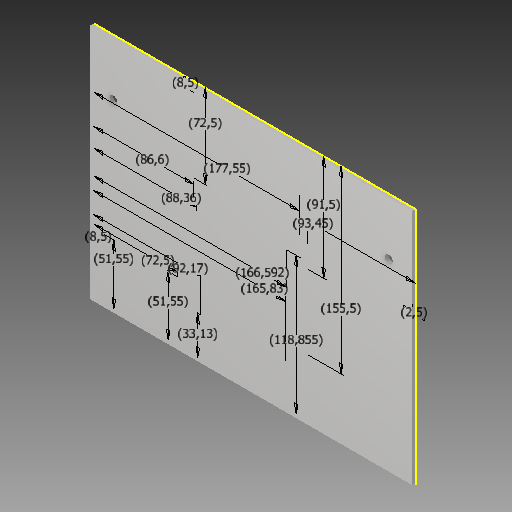
# Autodesk Inventor part: SupportsheetADCS2
Saved by Autodesk Inventor 2017 (Build 210142000, 142)
## iProperties
Created: 2016-11-08
Part Number: SupportsheetADCS2
Material: Aluminum 6061
Document SubType Name: Modeling
Designer: Jonis
Density: 2.7 g/cm^3
Appearance: Aluminum - Flat
Author: Jonis
Autodesk Inventor part; units mm, degrees
ref_plane "YZ Plane" through (0, 0, 0) normal (1, 0, 0) x (0, 1, 0)
ref_plane "XZ Plane" through (0, 0, 0) normal (0, 1, 0) x (-1, 0, 0)
ref_plane "XY Plane" through (0, 0, 0) normal (0, 0, 1) x (1, 0, 0)
sketch "Sketch1" plane through (0, 0, 0) normal (0, 0, 1) x (1, 0, 0)
  line L0 (0, 0) -> (278, 0)
  line L1 (278, 0) -> (278, 179)
  line L2 (278, 179) -> (0, 179)
  line L3 (0, 179) -> (0, 0)
  dimension "d0" = 278
  dimension "d1" = 179
  constraints: 8 end point, 2 parallel, 1 horizontal, 1 perpendicular
  measures "d0" distance of L2.end L1.end
  measures "d1" distance of L1.end L0.end
extrude "Extrusion1" add sketch "Sketch1" along normal blind 3
sketch "Sketch2" plane through (0, 0, 3) normal (0, 0, 1) x (1, 0, 0)
  line L0 (0, 179) -> (0, 0) projected
  line L1 (278, 179) -> (0, 179) projected
  line L2 (278, 0) -> (278, 179) projected
  point P0 (20, 159)
  point P1 (258, 159)
  dimension "d4" = 20
  dimension "d5" = 20
  dimension "d6" = 20
  dimension "d7" = 20
  measures "d4" distance from line of L0 point (20, 159)
  measures "d5" distance from line of L1 point (20, 159)
  measures "d6" distance from line of L1 point (258, 159)
  measures "d7" distance from line of L2 point (258, 159)
hole "Hole1" at (20, 159, 3) at (258, 159, 3) direction (0, 0, -1) diameter 7 end through all
sketch "Sketch6" plane through (0, 179, 0) normal (0, 1, 0) x (1, 0, 0)
  line L0 (0, 0) -> (278, 0) projected
  line L1 (0, -3) -> (278, -3) projected
  line L2 (0, 0) -> (278, 0)
  line L3 (278, 0) -> (278, -3)
  line L4 (278, -3) -> (0, -3)
  line L5 (0, -3) -> (0, 0)
  constraints: 8 end point, 2 parallel, 1 horizontal, 1 perpendicular
extrude "Extrusion2" add sketch "Sketch6" along normal blind 26
sketch "Sketch7" plane through (0, 0, 0) normal (0, 0, -1) x (-1, 0, 0)
  circle A0 centre (-92.17, 33.13) radius 1.5875 projected
  circle A1 centre (-165.83, 33.13) radius 1.5875 projected
  circle A2 centre (-166.592, 118.855) radius 1.5875 projected
  circle A3 centre (-88.36, 118.855) radius 1.5875 projected
  circle A4 centre (-8.5, 51.55) radius 1.6 projected
  circle A5 centre (-72.5, 51.55) radius 1.6 projected
  circle A6 centre (-72.5, 142.5) radius 1.6 projected
  circle A7 centre (-8.5, 142.5) radius 1.6 projected
  circle A8 centre (-86.6, 132.5) radius 1.6 projected
  circle A9 centre (-86.6, 196.5) radius 1.6 projected
  circle A10 centre (-177.55, 196.5) radius 1.6 projected
  circle A11 centre (-177.55, 132.5) radius 1.6 projected
  circle A12 centre (-184.55, 132.5) radius 1.6 projected
  circle A13 centre (-184.55, 196.5) radius 1.6 projected
  circle A14 centre (-275.5, 196.5) radius 1.6 projected
  circle A15 centre (-275.5, 132.5) radius 1.6 projected
  circle A16 centre (-275.5, 113.5) radius 1.6 projected
  circle A17 centre (-275.5, 49.5) radius 1.6 projected
  circle A18 centre (-184.55, 49.5) radius 1.6 projected
  circle A19 centre (-184.55, 113.5) radius 1.6 projected
  line L0 (0, 0) -> (-278, 0) projected
  line L1 (0, 0) -> (0, 205) projected
  line L2 (-278, 205) -> (0, 205) projected
  line L3 (-278, 0) -> (-278, 205) projected
  dimension "d41" = 33.13
  dimension "d42" = 51.55
  dimension "d43" = 51.55
  dimension "d44" = 8.5
  dimension "d45" = 72.5
  dimension "d46" = 88.36
  dimension "d47" = 92.17
  dimension "d48" = 165.83
  dimension "d49" = 166.592
  dimension "d50" = 86.6
  dimension "d51" = 177.55
  dimension "d52" = 8.5
  dimension "d53" = 72.5
  dimension "d54" = 2.5
  dimension "d55" = 93.45
  dimension "d56" = 91.5
  dimension "d57" = 155.5
  dimension "d58" = 118.855
  measures "d41" distance from line of A0.centre L0
  measures "d42" distance from line of A5.centre L0
  measures "d43" distance from line of A4.centre L0
  measures "d44" distance from line of A4.centre L1
  measures "d45" distance from line of A5.centre L1
  measures "d46" distance from line of A3.centre L1
  measures "d47" distance from line of A0.centre L1
  measures "d48" distance from line of A1.centre L1
  measures "d49" distance from line of A2.centre L1
  measures "d50" distance from line of A8.centre L1
  measures "d51" distance from line of A11.centre L1
  measures "d52" distance from line of A9.centre L2
  measures "d53" distance from line of A8.centre L2
  measures "d54" distance from line of A15.centre L3
  measures "d55" distance from line of A12.centre L3
  measures "d56" distance from line of L2 A19.centre
  measures "d57" distance from line of A18.centre L2
  measures "d58" distance from line of A2.centre L0
body "Solid1"
